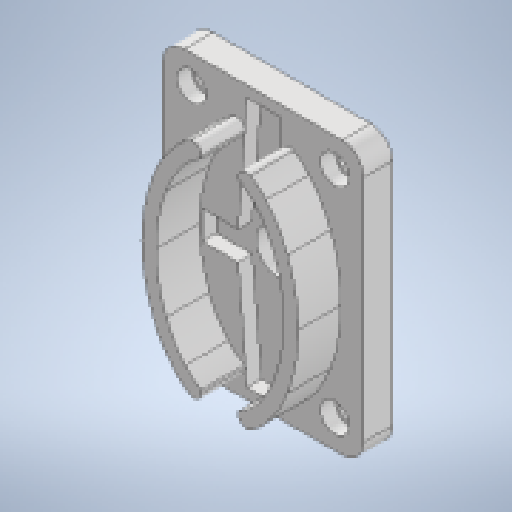
# Autodesk Inventor part: base
Saved by Autodesk Inventor 2024 (Build 280153000, 153)
## iProperties
Created: 2025-05-13
Part Number: base
Material: Genérico
Document SubType Name: Modeling
Designer: mario
Density: 1 g/cm^3
Appearance: Valor por defecto
Author: mario
Autodesk Inventor part; units mm, degrees
ref_plane "YZ Plane" through (0, 0, 0) normal (1, 0, 0) x (0, 1, 0)
ref_plane "XZ Plane" through (0, 0, 0) normal (0, 1, 0) x (-1, 0, 0)
sketch "Boceto5" plane through (-24, -1, 0) normal (0, 0, -1) x (-1, 0, 0)
  line L0 (-28, 35) -> (0, 35)
  line L1 (0, 35) -> (0, -3)
  line L2 (0, -3) -> (-28, -3)
  line L3 (-28, -3) -> (-28, 35)
  point P0 (-24, 1)
  point P1 (0, 0)
  dimension "d3" = 28
  dimension "d4" = 3
  dimension "d5" = 35
  constraints: 8 end point, 2 parallel, 1 horizontal, 1 perpendicular, 1 point on line
  measures "d3" distance between parallel lines of L1 L3
  measures "d4" distance from line of point (0, 0) L2
  measures "d5" distance from line of point (0, 0) L0
extrude "Extrusión2" add sketch "Boceto5" against normal blind 4
fillet "Empalme1" radius 3 4 edges at (-24, -4, 2) (4, -4, 2) (4, 34, 2) (-24, 34, 2)
sketch "Boceto6" plane through (-24, -1, 4) normal (0, 0, 1) x (1, 0, 0)
  line L0 (25, 35) -> (3, 35) construction
  line L1 (0, 32) -> (0, 0) construction
  point P0 (24, 1)
  point P1 (4, 31)
  dimension "d9" = 4
  dimension "d10" = 4
  measures "d9" distance from line of L0 point (4, 31)
  measures "d10" distance from line of point (4, 31) L1
hole "Agujero1" at (-20, 30, 4) direction (0, 0, -1) diameter 3 end through all counterbore diameter 4 counterbore depth 2
pattern_linear "Patrón rectangular1" count 2 spacing 20 along (1, 0, 0) count 2 spacing 30 along (0, -1, 0) of "Agujero1"
sketch "Boceto7" plane through (-24, -1, 0) normal (0, 0, -1) x (-1, 0, 0)
  line L0 (-3, 35) -> (-25, 35) projected
  line L1 (-28, 32) -> (-28, 0) projected
  point P0 (-24, 1)
  point P1 (-14, 15)
  dimension "d24" = 20
  dimension "d25" = 14
  measures "d24" distance from line of L0 point (-14, 15)
  measures "d25" distance from line of L1 point (-14, 15)
hole "Agujero2" at (-10, 14, 0) direction (0, 0, 1) diameter 6 end through all
sketch "Boceto8" plane through (-24, -1, 4) normal (0, 0, 1) x (1, 0, 0)
  line L0 (5.5, 17) -> (22.5, 17)
  line L1 (22.5, 17) -> (22.5, 13)
  line L2 (22.5, 13) -> (5.5, 13)
  line L3 (5.5, 13) -> (5.5, 17)
  circle A0 centre (14, 15) radius 3 projected
  line L4 (5.5, 17) -> (22.5, 13) construction
  line L5 (22.5, 17) -> (5.5, 13) construction
  point P0 (24, 1)
  point P1 (11.7639, 13)
  point P2 (11.7639, 17)
  point P3 (16.2361, 17)
  point P4 (16.2361, 13)
  dimension "d33" = 17
  dimension "d34" = 4
  constraints: 12 end point, 2 midpoint, 2 parallel, 1 horizontal, 1 perpendicular
  measures "d33" distance of L1.end L2.end
  measures "d34" distance of L0.end L1.end
extrude "Extrusión3" cut sketch "Boceto8" against normal blind 2 contours L0 A0 L2 L3 | L0 L1 L2 A0
sketch "Boceto9" plane through (-24, -1, 4) normal (0, 0, 1) x (1, 0, 0)
  line L0 (11.7639, 13) -> (5.5, 13) construction
  line L1 (10.5, 13) -> (11.75, -1.5)
  line L2 (11.75, -1.5) -> (16.25, -1.5)
  line L3 (16.25, -1.5) -> (17.5, 13)
  line L4 (17.5, 13) -> (10.5, 13)
  line L5 (0, 32) -> (0, 0) projected
  point P0 (24, 1)
  dimension "d37" = 14.5
  dimension "d38" = 4.5
  dimension "d39" = 10.5
  dimension "d40" = 7
  dimension "d41" = 1.25
  constraints: 8 end point, 2 horizontal, 1 point on line
  measures "d37" distance between parallel lines of L2 L4
  measures "d38" distance of L1.end L2.end
  measures "d39" distance from line of L5 L1.start
  measures "d40" distance of L3.end L1.start
  measures "d41" horizontal distance of L1.end L1.start
extrude "Extrusión4" cut sketch "Boceto9" against normal blind 2
sketch "Boceto11" plane through (-24, -1, 4) normal (0, 0, 1) x (1, 0, 0)
  line L0 (5.5, 17) -> (11.7639, 17) construction
  line L1 (10.5, 17) -> (17.5, 17)
  line L2 (17.5, 17) -> (16.25, 33.5)
  line L3 (16.25, 33.5) -> (11.75, 33.5)
  line L4 (11.75, 33.5) -> (10.5, 17)
  point P0 (24, 1)
  dimension "d44" = 16.5
  dimension "d46" = 5
  dimension "d47" = 1.25
  dimension "d48" = 7
  constraints: 8 end point, 2 horizontal, 1 equal length, 1 point on line
  measures "d44" distance between parallel lines of L1 L3
  measures "d46" distance of L0.start L1.start
  measures "d47" horizontal distance of L1.start L3.end
  measures "d48" distance of L1.start L1.end
extrude "Extrusión5" cut sketch "Boceto11" against normal blind 2
sketch "Boceto15" plane through (-13.8306, 0.9703, 10) normal (0, 0, 1) x (1, 0, 0)
  circle A0 centre (17.3236, 13.0832) radius 22.3484 construction
  circle A1 centre (4.7289, 20.1353) radius 7.5795 construction
  circle A2 centre (10.4075, 15.4052) radius 15.0152 construction
  arc A3 (-3.6953, 20.6765) -> (-5.0248, 13.0297) centre (17.3236, 13.0832) ccw
  arc A4 (-1.0419, 25.1821) -> (-3.6953, 20.6765) centre (10.4075, 15.4052) ccw
  arc A5 (1.2391, 26.9612) -> (-1.0419, 25.1821) centre (4.7289, 20.1353) ccw
  circle A6 centre (3.8306, 13.0297) radius 3 construction
  line L0 (3.8306, 13.0297) -> (-5.0248, 13.0297) construction
  line L1 (3.8306, 11.0151) -> (-6.9515, 11.0151) construction
  arc A7 (-5.5863, 21.3713) -> (-6.9515, 11.0151) centre (17.3236, 13.0832) ccw
  arc A8 (-2.5664, 26.4991) -> (-5.5863, 21.3713) centre (10.4075, 15.4052) ccw
  arc A9 (-0.3913, 28.3513) -> (-2.5664, 26.4991) centre (4.7289, 20.1353) ccw
  line L2 (0.3306, 15.0297) -> (1.5806, 31.5297) construction
  arc A10 (1.2648, 27.3612) -> (-0.3913, 28.3513) centre (0.1824, 27.4308) ccw
  line L3 (1.2648, 27.3612) -> (1.2391, 26.9612)
  arc A11 (-5.0248, 13.0297) -> (-3.6953, 5.3829) centre (17.3236, 12.9762) ccw
  arc A12 (-3.6953, 5.3829) -> (-1.0419, 0.8774) centre (10.4075, 10.6542) ccw
  arc A13 (-1.0419, 0.8774) -> (1.2391, -0.9018) centre (4.7289, 5.9242) ccw
  line L4 (3.8306, 15.0443) -> (-6.9515, 15.0443) construction
  arc A14 (-6.9515, 15.0443) -> (-5.5863, 4.6881) centre (17.3236, 12.9762) ccw
  arc A15 (-5.5863, 4.6881) -> (-2.5664, -0.4397) centre (10.4075, 10.6542) ccw
  arc A16 (-2.5664, -0.4397) -> (-0.3913, -2.2919) centre (4.7289, 5.9242) ccw
  arc A17 (-0.3913, -2.2919) -> (1.2648, -1.3018) centre (0.1824, -1.3713) ccw
  line L5 (1.2648, -1.3018) -> (1.2391, -0.9018)
  point P0 (13.8306, -0.9703)
  point P1 (0.3306, 11.0297)
  point P2 (-7.0394, 13.0297)
  dimension "d51" = 20
  dimension "d52" = 20
  dimension "d53" = 21.75
  dimension "d55" = 1.9267
  dimension "d56" = 0.4
  constraints: 28 point on circle, 15 symmetric about line, 14 centre point, 10 end point, 4 coincident, 2 tangent, 1 horizontal, 1 point on line, 14 other
  measures "d55" horizontal distance of L0.end L1.end
  measures "d56" vertical distance of L3.start L3.end
extrude "Extrusión6" add sketch "Boceto15" against normal blind 6
ref_plane "Plano de trabajo2" through (-10, 12, 4) normal (1, 0, 0) x (0, 0, -1)
mirror "Simetría2" about plane through (-10, 12, 4) normal (1, 0, 0) of "Extrusión6"
